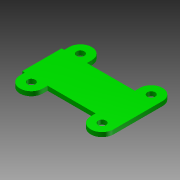
# Autodesk Inventor part: BatteryLatch-Lower
Saved by Autodesk Inventor 2012 (Build 160160000, 160)
## iProperties
Created: 2013-10-13
Part Number: BatteryLatch-Lower
Material: Default
Document SubType Name: Modeling
Designer: joe_000
Density: 1 g/cm^3
Author: joe_000
Autodesk Inventor part; units mm, degrees
ref_plane "YZ Plane" through (0, 0, 0) normal (1, 0, 0) x (0, 1, 0)
ref_plane "XZ Plane" through (0, 0, 0) normal (0, 1, 0) x (-1, 0, 0)
ref_plane "XY Plane" through (0, 0, 0) normal (0, 0, 1) x (1, 0, 0)
sketch "Sketch1" plane through (0, 0, 0) normal (0, 1, 0) x (-1, 0, 0)
  line L0 (0, 0) -> (-34.925, 0)
  line L1 (-34.925, 0) -> (-34.925, -14.2875)
  line L2 (-34.925, -14.2875) -> (0, -14.2875)
  line L3 (0, -14.2875) -> (0, 0)
  line L4 (-34.925, 0) -> (-34.925, 1.778)
  line L5 (-26.6438, 0) -> (-26.6438, 1.778)
  arc A0 (-26.6438, 1.778) -> (-34.925, 1.778) centre (-30.7844, 1.778) ccw
  circle A1 centre (-30.7844, 1.778) radius 1.4224
  line L6 (-9.2075, 0) -> (-9.2075, 1.778)
  line L7 (-0.9263, 0) -> (-0.9263, 1.778)
  arc A2 (-0.9263, 1.778) -> (-9.2075, 1.778) centre (-5.0669, 1.778) ccw
  circle A3 centre (-5.0669, 1.778) radius 1.4224
  line L8 (-34.925, -7.1437) -> (0, -7.1437)
  line L9 (-34.925, -14.2875) -> (-34.925, -16.0655)
  line L10 (-26.6438, -14.2875) -> (-26.6438, -16.0655)
  arc A4 (-34.925, -16.0655) -> (-26.6438, -16.0655) centre (-30.7844, -16.0655) ccw
  circle A5 centre (-30.7844, -16.0655) radius 1.4224
  arc A6 (-9.2075, -16.0655) -> (-0.9263, -16.0655) centre (-5.0669, -16.0655) ccw
  line L11 (-0.9263, -14.2875) -> (-0.9263, -16.0655)
  line L12 (-9.2075, -14.2875) -> (-9.2075, -16.0655)
  circle A7 centre (-5.0669, -16.0655) radius 1.4224
  line L13 (-9.2075, 0) -> (-0.9263, 0)
  line L14 (-0.9263, -14.2875) -> (-9.2075, -14.2875)
  line L15 (-26.6438, -14.2875) -> (-34.925, -14.2875)
  dimension "d2" = 34.925
  dimension "d3" = 14.2875
  dimension "d5" = 1.778
  dimension "d6" = 8.2812
  dimension "d8" = 2.8448
  dimension "d11" = 25.7175
  constraints: 32 end point, 12 symmetric about line, 8 centre point, 8 point on circle, 4 coincident, 4 parallel, 3 collinear, 2 horizontal, 2 midpoint, 2 perpendicular, 2 point on line, 2 tangent, 14 other
  measures "d2" distance of L0.start L0.end
  measures "d3" distance of L0.end L1.end
  measures "d5" distance of L4.start L4.end
  measures "d6" distance between parallel lines of L5 L4
  measures "d8" diameter of A1
  measures "d11" distance of A0.centre A2.centre
extrude "Extrusion1" add sketch "Sketch1" along normal blind 1.5875
equation "\"d2\" = outerLength + wallThickness"
equation "\"d3\" = outerWidth"
equation "\"d5\" = screwHoleOffsetFromSide"
equation "\"d6\" = screwOuterDiameter"
equation "\"d0\" = wallThickness"
equation "\"outerLength\" = 33.3375"
equation "\"wallThickness\" = 1.5875"
equation "\"outerWidth\" = 14.2875"
equation "\"screwHoleOffsetFromSide\" = 1.778"
equation "\"screwOuterDiameter\" = 8.281182"
body "Solid1"
